Autodesk Inventor part; units mm, degrees
note: some values were not read from the file. Chosen so that the rebuilt part matches the saved one: direction of "Hole2".
(part 18 of 18)
sketch "Sketch18" plane through (0, 13.762, -7.5) normal (0, 1, 0) x (1, 0, 0)
  line L0 (-9.984, -8.484) -> (-9.984, 31.4609) projected
  line L1 (-9.984, 31.4609) -> (9.984, 31.4609) projected
  line L2 (9.984, 31.4609) -> (9.984, -8.484) projected
  line L3 (9.984, -8.484) -> (-9.984, -8.484) projected
  line L4 (11, -9.5) -> (11, 32.4769) projected
  line L5 (11, 32.4769) -> (-11, 32.4769) projected
  line L6 (-11, 32.4769) -> (-11, -9.5) projected
  line L7 (-11, -9.5) -> (11, -9.5) projected
  point P0 (0, -7.5)
  point P1 (-9.984, -7.5)
  point P2 (9.984, -7.5)
extrude "Extrusion13" add sketch "Sketch18" along normal blind 12 draft 6
sketch "Sketch19" plane through (0, 25.762, -7.5) normal (0, 1, 0) x (1, 0, 0)
  line L0 (-10.7373, 31.7382) -> (10.527, 31.7382)
  line L1 (10.527, 31.7382) -> (10.527, -9.2373)
  line L2 (10.527, -9.2373) -> (-10.7373, -9.2373)
  line L3 (-10.7373, -9.2373) -> (-10.7373, 31.7382)
  line L4 (-12.2613, 33.7382) -> (12.2613, 33.7382) projected
  line L5 (12.2613, -10.7613) -> (-12.2613, -10.7613) projected
  line L6 (-12.2613, -10.7613) -> (-12.2613, 33.7382) projected
  point P0 (0, -7.5)
  point P1 (-0.1051, 31.7382)
  point P2 (-0.1051, 30.8661)
  dimension "d183" = 2
  dimension "d184" = 1.524
  dimension "d185" = 1.524
  constraints: 8 end point, 2 parallel, 1 horizontal, 1 midpoint, 1 perpendicular, 1 vertical alignment
  measures "d183" distance between parallel lines of L0 L4
  measures "d184" distance between parallel lines of L5 L2
  measures "d185" distance between parallel lines of L3 L6
sketch "Sketch20" plane through (0, 13.762, -7.5) normal (0, 1, 0) x (-1, 0, 0)
  line L0 (9.984, 8.484) -> (-9.984, 8.484)
  line L1 (-9.984, 8.484) -> (-9.984, -31.4609)
  line L2 (-9.984, -31.4609) -> (9.984, -31.4609)
  line L3 (9.984, -31.4609) -> (9.984, 8.484)
  point P0 (0, 7.5)
  constraints: 8 end point, 2 parallel, 1 coincident, 1 horizontal, 1 perpendicular
loft "Loft1" cut profiles "Sketch20", "Sketch19"
ref_plane "Work Plane11" through (0, 0, -53) normal (0, 0, -1) x (-1, 0, 0)
sketch "Sketch71" plane through (0, 25.762, -41.2382) normal (0, 0.9876883, 0.1564345) x (1, 0, 0)
  line L0 (-21.5783, 4.8479) -> (20.8783, 4.8479)
  line L1 (20.8783, 4.8479) -> (20.8783, -47.9416)
  line L2 (20.8783, -47.9416) -> (-21.5783, -47.9416)
  line L3 (-21.5783, -47.9416) -> (-21.5783, 4.8479)
  point P0 (0, 0)
  constraints: 8 end point, 2 parallel, 1 horizontal, 1 perpendicular
extrude "Extrusion27" cut sketch "Sketch71" along normal through all
equation "\"d22\" = d24"
equation "\"d23\" = d24"
equation "\"d37\" = t"
equation "\"d40\" = t"
equation "\"t\" = 1.016"
equation "\"d14\" = d24"
equation "\"d24\" = 1.016"
body "Solid1"
